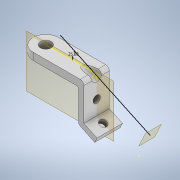
# Autodesk Inventor part: 3번
Saved by Autodesk Inventor 2022 (Build 260153000, 153)
## iProperties
Created: 2021-09-04
Part Number: 3번
Material: 일반
Document SubType Name: Modeling
Designer: 서울공업고등학교
Density: 1 g/cm^3
Appearance: 기본값
Author: 서울공업고등학교
Autodesk Inventor part; units mm, degrees
ref_plane "YZ Plane" through (0, 0, 0) normal (1, 0, 0) x (0, 1, 0)
ref_plane "XZ Plane" through (0, 0, 0) normal (0, 1, 0) x (-1, 0, 0)
ref_plane "XY Plane" through (0, 0, 0) normal (0, 0, 1) x (1, 0, 0)
sketch "스케치1" plane through (0, 0, 0) normal (0, 0, 1) x (1, 0, 0)
  line L0 (0, 0) -> (0, -10)
  line L1 (0, -10) -> (80, -10)
  line L2 (80, -10) -> (80, -54.778)
  line L3 (80, -54.778) -> (102.4565, -65.2497)
  line L4 (102.4565, -65.2497) -> (105.6262, -58.4524)
  line L5 (105.6262, -58.4524) -> (87.5, -50)
  line L6 (87.5, -50) -> (87.5, 0)
  line L7 (87.5, 0) -> (0, 0)
  dimension "d5" = 7.5
  dimension "d7" = 20
  dimension "d9" = 7.5
  dimension "d10" = 50
  dimension "d11" = 10
  dimension "d12" = 115
  dimension "d13" = 87.5
  constraints: 16 end point, 4 perpendicular, 1 horizontal, 1 parallel, 1 vertical
  measures "d5" distance of L3.end L4.end
  measures "d7" distance of L4.end L5.end
  measures "d9" distance between parallel lines of L6 L2
  measures "d10" distance of L6.end L5.end
  measures "d11" distance between parallel lines of L1 L7
  measures "d12" angle of L5 L6
  measures "d13" distance between parallel lines of L6 L0
extrude "돌출1" add sketch "스케치1" along normal mid plane 35
fillet "모깎기1" radius 17.5 1 edges at (0, -5, -17.5)
fillet "모깎기2" radius 17.5 1 edges at (0, -5, 17.5)
fillet "모깎기3" radius 2 1 edges at (80, -10, 0)
fillet "모깎기5" radius 5 1 edges at (80, -54.778, 0)
sketch "스케치3" plane through (87.5, 0, 17.5) normal (0, 1, 0) x (1, 0, 0)
  arc A0 (-70, 35) -> (-70, 0) centre (-70, 17.5) ccw projected
  circle A1 centre (-70, 17.5) radius 7.5
  point P0 (-87.5, 17.5)
  dimension "d22" = 15
  constraints: 1 centre point, 1 coincident
  measures "d22" diameter of A1
sketch "스케치4" plane through (87.5, -50, 17.5) normal (0.4226183, 0.9063078, 0) x (0.9063078, -0.4226183, 0)
  circle A0 centre (10, 17.5) radius 5
  line L0 (0, 35) -> (0, 0) projected
  point P0 (-100.4328, 17.5)
  dimension "d23" = 10
  dimension "d24" = 10
  constraints: 1 centre point
  measures "d23" diameter of A0
  measures "d24" distance from line of A0.centre L0
ref_plane "작업 평면1" through (0, 0, 0) normal (0, 0, 1) x (1, 0, 0)
fillet "모깎기7" radius 5 1 edges at (87.5, 0, 0)
sketch "스케치6" plane through (0, 0, 0) normal (0, 0, 1) x (1, 0, 0)
  line L0 (37.61, 21.4494) -> (161.1108, -36.1399)
  arc A0 (87.5, -5) -> (82.5, 0) centre (82.5, -5) ccw projected
  line L1 (17.5, 0) -> (82.5, 0) projected
  point P0 (0, 0)
  dimension "d26" = 25
  constraints: 2 end point, 1 tangent
  measures "d26" angle of L1 L0
ref_plane "작업 평면2" through (161.1108, -36.1399, 0) normal (0.9063078, -0.4226183, 0) x (0.4226183, 0.9063078, 0)
sketch "스케치7" plane through (161.1108, -36.1399, 0) normal (0.9063078, -0.4226183, 0) x (0.4226183, 0.9063078, 0)
  point P0 (-35.3345, 0)
sketch "스케치8" plane through (161.1108, -36.1399, 0) normal (0.9063078, -0.4226183, 0) x (0.4226183, 0.9063078, 0)
  point P0 (-35.3345, 0)
sketch "스케치9" plane through (161.1108, -36.1399, 0) normal (0.9063078, -0.4226183, 0) x (0.4226183, 0.9063078, 0)
  line L0 (0, -17.5) -> (0, 17.5) projected
  circle A0 centre (0, 0) radius 7
  point P0 (-35.3345, 0)
  dimension "d27" = 14
  constraints: 1 centre point, 1 midpoint
  measures "d27" diameter of A0
extrude "돌출2" cut sketch "스케치9" against normal blind 200
extrude "돌출3" cut sketch "스케치3" against normal blind 200
extrude "돌출4" cut sketch "스케치4" against normal blind 200
sketch "스케치10" plane through (87.5, -50, 17.5) normal (1, 0, 0) x (0, 0, -1)
  circle A0 centre (17.5, 20) radius 5
  line L0 (10.5157, 50) -> (24.4843, 50) projected
  point P0 (17.5, 50)
  dimension "d34" = 10
  dimension "d35" = 30
  constraints: 1 centre point
  measures "d34" diameter of A0
  measures "d35" distance from line of A0.centre L0
extrude "돌출5" cut sketch "스케치10" against normal blind 60
